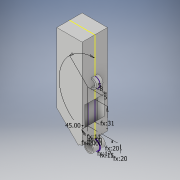
# Autodesk Inventor part: lower leg V2
Saved by Autodesk Inventor 2019 (Build 230136000, 136)
## iProperties
Created: 2018-07-06
Part Number: lower leg V2
Material: Generic
Document SubType Name: Modeling
Designer: HIVE
Density: 1 g/cm^3
Appearance: Default
Author: HIVE
Autodesk Inventor part; units mm, degrees
ref_plane "YZ Plane" through (0, 0, 0) normal (1, 0, 0) x (0, 1, 0)
ref_plane "XZ Plane" through (0, 0, 0) normal (0, 1, 0) x (-1, 0, 0)
ref_plane "XY Plane" through (0, 0, 0) normal (0, 0, 1) x (1, 0, 0)
sketch "Sketch1" plane through (0, 0, 0) normal (0, 1, 0) x (-1, 0, 0)
  line L0 (0, 0) -> (40, 0)
  line L1 (40, 0) -> (40, -40)
  line L2 (40, -40) -> (0, -40)
  line L3 (0, -40) -> (0, 0)
  dimension "d9" = 40
  dimension "d10" = 40
  constraints: 8 end point, 2 parallel, 1 horizontal, 1 perpendicular
  measures "d9" distance of L1.end L2.end
  measures "d10" distance of L0.end L1.end
extrude "Extrusion1" add sketch "Sketch1" along normal blind 150
ref_plane "Work Plane1" through (-40, 0, -20) normal (0, 0, 1) x (1, 0, 0)
sketch "Sketch2" plane through (-40, 0, -20) normal (0, 0, 1) x (1, 0, 0)
  line L0 (40, 0) -> (0, 0) projected
  line L1 (40, 0) -> (40, 150) projected
  line L2 (0, 150) -> (40, 150) projected
  line L3 (0, 0) -> (0, 150) projected
  line L4 (40, 31) -> (29, 20)
  line L5 (29, 20) -> (29, 73)
  line L6 (29, 73) -> (40, 62)
  line L7 (40, 0) -> (40, 150) projected
  arc A0 (40, 81) -> (40, 91) centre (40, 86) ccw
  arc A1 (40, 78) -> (40, 94) centre (40, 86) ccw
  line L8 (0, 0) -> (40, 0) projected
  line L9 (40, 0) -> (0, 0) projected
  line L10 (40, 0) -> (20, 0)
  line L11 (20, 0) -> (20, 0)
  line L12 (20, 0) -> (40, 0)
  line L13 (40, 0) -> (40, 0)
  line L14 (40, 31) -> (40, 62)
  circle A2 centre (40, 0) radius 5.5
  arc A3 (32.5, 0) -> (34.6967, 5.3033) centre (40, 0) ccw
  arc A4 (31.5, 0) -> (33.9896, 6.0104) centre (40, 0) ccw
  arc A5 (33.9896, 6.0104) -> (31.5, 0) centre (40, 0) ccw
  line L15 (31.5, 0) -> (0, 0)
  line L16 (0, 0) -> (0, 150) projected
  line L17 (0, 40) -> (0, 0)
  line L18 (0, 40) -> (34.6967, 5.3033)
  arc A6 (34.6967, 5.3033) -> (32.5, 0) centre (40, 0) ccw
  dimension "d2" = 45
  dimension "d3" = 45
  dimension "d5" = 11
  dimension "d8" = 31
  dimension "d12" = 5
  dimension "d13" = 8
  dimension "d14" = 5
  dimension "d28" = 20
  dimension "d30" = 20
  dimension "d35" = 20
  dimension "d36" = 11
  dimension "d37" = 15
  dimension "d38" = 17
  dimension "d42" = 45
  constraints: 22 end point, 12 point on circle, 10 point on line, 7 centre point, 3 coincident, 2 collinear, 2 vertical, 1 horizontal, 1 parallel, 1 perpendicular
  measures "d2" angle of L1 L6
  measures "d3" angle of L1 L4
  measures "d5" distance between parallel lines of L1 L5
  measures "d8" distance of L4.start L6.end
  measures "d12" vertical distance of L5.end A1.start
  measures "d13" radius of A1
  measures "d14" radius of A0
  measures "d28" distance of L12.end L11.end
  measures "d30" distance from line of L12 L4.end
  measures "d35" distance from line of L0 L4.end
  measures "d36" diameter of A2
  measures "d37" diameter of A3
  measures "d38" diameter of A4
  measures "d42" angle of L3 L18
extrude "Extrusion3" add sketch "Sketch2" along normal mid plane 10 contours L1 A0 A1
extrude "Extrusion4" add sketch "Sketch2" along normal mid plane 18 contours A6 A3 L1 A2 L0 | L0 A2 L1 A3
extrude "Extrusion5" cut sketch "Sketch2" along normal through all both and the other way through all contours A2 L1 L0 | L0 L1 A2
extrude "Extrusion6" cut sketch "Sketch2" along normal up to surface (11 mm away) from surface at 9 contours A3 L1 A4 L0 | A6 A3 L1 A2 L0 | L0 A2 L1 A3 | L0 A5 L18 A6 | A3 L18 A4 L1
extrude "Extrusion7" cut sketch "Sketch2" against normal up to surface (11 mm away) from surface at -9 contours A3 L1 A4 L0 | A6 A3 L1 A2 L0 | L0 A2 L1 A3 | L0 A5 L18 A6 | A3 L18 A4 L1
extrude "Extrusion8" cut sketch "Sketch2" along normal mid plane 31 contours L4 L5 L6 L1
extrude "Extrusion11" cut sketch "Sketch2" along normal mid plane 40 contours L0 A5 L18 A6 | L0 L3 L18 A5
equation "\"d9\" = legDiam"
equation "\"d10\" = legDiam"
equation "\"d5\" = kneeBallBaseH + clearance"
equation "\"d8\" = kneeBallBaseW + clearance"
equation "\"d28\" = kneeBallDepth"
equation "\"d30\" = kneeBallLocationExtend"
equation "\"d35\" = kneeBallLocationExtend"
equation "\"d36\" = kneeBallBaseH + clearance"
equation "\"d19\" = 0.5 * legDiam - 2 * clearance"
equation "\"d31\" = kneeBallBaseW + clearance"
equation "\"d43\" = legDiam"
equation "\"legDiam\" = 40"
equation "\"kneeBallBaseH\" = 10"
equation "\"clearance\" = 1"
equation "\"kneeBallBaseW\" = 30"
equation "\"kneeBallDepth\" = 20"
equation "\"kneeBallLocationExtend\" = 20"
body "Solid1"
